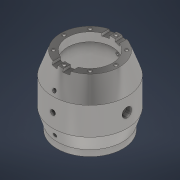
# Autodesk Inventor part: Emitter_Barrel
Saved by Autodesk Inventor 2022 (Build 260153000, 153)
## iProperties
Created: 2024-05-08
Part Number: Emitter_Barrel
Material: Generic
Document SubType Name: Modeling
Designer: jo_ki
Density: 1 g/cm^3
Appearance: Steel - Polished
Author: jo_ki
Autodesk Inventor part; units mm, degrees
sketch "Sketch1" plane through (0, 0, 0) normal (0, 0, 1) x (1, 0, 0)
  line L0 (0, 48) -> (0, -8) projected
  line L1 (0, 0) -> (19, 0)
  line L2 (19, 0) -> (19, 3.5)
  line L3 (19, 3.5) -> (21.5, 11.5)
  line L4 (21.5, 11.5) -> (21.5, 27.5)
  line L5 (21.5, 27.5) -> (17, 40)
  line L6 (17, 40) -> (13, 40)
  line L7 (13, 40) -> (13, 0)
  line L8 (-4.3, 0) -> (25.8, 0) construction
  line L9 (5.125, 40) -> (1.625, 40)
  line L10 (1.625, 40) -> (1.625, 38.5)
  line L11 (1.625, 38.5) -> (5.125, 38.5)
  line L12 (5.125, 38.5) -> (5.125, 40)
  line L13 (13, 35) -> (16, 35)
  line L14 (16, 35) -> (16, 0)
  line L15 (14, 40) -> (14, 0)
  point P0 (16, 0)
  dimension "d0" = 38
  dimension "d1" = 3.5
  dimension "d2" = 43
  dimension "d3" = 11.5
  dimension "d5" = 34
  dimension "d6" = 40
  dimension "d7" = 26
  dimension "d9" = 3.5
  dimension "d10" = 1.5
  dimension "d11" = 3.25
  dimension "d24" = 32
  dimension "d56" = 27.5
  dimension "d57" = 5
  dimension "d59" = 2
  constraints: 28 end point, 5 perpendicular, 5 point on line, 4 parallel, 3 horizontal, 1 collinear
  measures "d0" diameter of L1.end L0
  measures "d1" distance from line of L2.end L8
  measures "d2" diameter of L3.end L0
  measures "d3" distance from line of L8 L3.end
  measures "d5" diameter of L5.end L0
  measures "d6" distance from line of L8 L5.end
  measures "d7" diameter of L6.end L0
  measures "d9" distance between parallel lines of L10 L12
  measures "d10" distance between parallel lines of L11 L9
  measures "d11" diameter of L10 L0
  measures "d24" diameter of L14 L0
  measures "d56" distance from line of L8 L4.end
  measures "d57" distance between parallel lines of L13 L6
  measures "d59" distance between parallel lines of L15 L14
revolve "Revolution1" add sketch "Sketch1" angle 360 about axis through (0, 0, 0) along (0, -1, 0) contours L7 L6 L15 L13 | L14 L13 L15 L6 L5 L4 L3 L2 L1
extrude "Extrusion1" cut sketch "Sketch1" along normal through all both and the other way through all contours L12 L11 L10 L9
mirror "Mirror1" about plane through (0, 0, 0) normal (1, 0, 0) of "Extrusion1"
sketch "Sketch4" plane through (1.625, 40, 16.9222) normal (0, 1, 0) x (1, 0, 0)
  line L0 (-3.25, 4.0241) -> (-3.25, 0) projected
  arc A0 (-3.25, 0) -> (0, 0) centre (-1.625, 16.9222) ccw projected
  line L1 (0, 0) -> (0, 4.0241) projected
  arc A1 (-3.25, 4.0241) -> (0, 4.0241) centre (-1.625, 16.9222) ccw projected
  line L2 (-1.625, 3.9222) -> (-1.625, -0.0778)
  line L3 (0, 29.8202) -> (0, 33.8443) projected
  line L4 (-3.25, 33.8443) -> (-3.25, 29.8202) projected
  arc A2 (0, 33.8443) -> (-3.25, 33.8443) centre (-1.625, 16.9222) ccw projected
  arc A3 (-3.25, 4.0241) -> (0, 4.0241) centre (-1.625, 16.9222) ccw projected
  arc A4 (0, 29.8202) -> (-3.25, 29.8202) centre (-1.625, 16.9222) ccw projected
  point P0 (-1.625, 1.9222)
  constraints: 2 end point, 2 point on circle, 1 midpoint
hole "Hole1" at (0, 40, 15) direction (0, -1, 0) diameter 2 depth 0.5 tip angle 118
pattern_circular "Circular Pattern1" count 8 over 360 about axis through (0, -10, 0) along (0, 1, 0) of "Hole1"
ref_plane "Work Plane1" through (0, 19.5, 21.5) normal (0, 0, 1) x (1, 0, 0)
sketch "Sketch5" plane through (0, 19.5, 21.5) normal (0, 0, 1) x (1, 0, 0)
  line L0 (-21.5, 8) -> (21.5, 8) projected
  line L1 (-21.5, -8) -> (21.5, -8) projected
  line L2 (-21.5, -8) -> (21.5, -8) projected
  line L3 (-21.5, 8) -> (21.5, 8) projected
  line L4 (0, 8) -> (0, -8)
  point P0 (0, -19.5)
  point P1 (0, 0)
  constraints: 3 midpoint, 2 end point
hole "Hole2" at (0, 19.5, 21.5) direction (0, 0, -1) diameter 2.9 depth 7.6 clearance for "Countersunk Flat Head Screw ISO 2009/7046" size "M2.5" standard "ISO"
ref_plane "Work Plane2" through (21.5, 19.5, 0) normal (1, 0, 0) x (0, 1, 0)
sketch "Sketch6" plane through (21.5, 19.5, 0) normal (1, 0, 0) x (0, 1, 0)
  line L0 (8, 21.5) -> (8, -21.5) projected
  line L1 (-8, 21.5) -> (-8, -21.5) projected
  line L2 (8, 0) -> (-8, 0)
  point P0 (-19.5, 0)
  point P1 (0, 0)
  constraints: 3 midpoint, 2 end point
hole "Hole3" at (21.5, 19.5, 0) direction (-1, 0, 0) diameter 2.9 depth 10 counterbore diameter 5.5 counterbore depth 2.9 clearance for "Socket Head Cap Screw DIN EN ISO 4762" size "M2.5" standard "DIN"
mirror "Mirror2" about plane through (0, 0, 0) normal (1, 0, 0) of "Hole3"
ref_plane "Work Plane3" through (0, 19.5, 21.5) normal (0, 0, 1) x (1, 0, 0)
sketch "Sketch7" plane through (0, 19.5, 21.5) normal (0, 0, 1) x (1, 0, 0)
  line L0 (-21.5, -8) -> (21.5, -8) projected
  line L1 (-19, -16) -> (19, -16) projected
  line L2 (-21.5, -8) -> (21.5, -8) projected
  line L3 (0, -8) -> (0, -16)
  line L4 (-21.5, 8) -> (21.5, 8) projected
  line L5 (-1.625, 20.5) -> (-1.625, 19) projected
  line L6 (-1.625, 19) -> (-5.125, 19) projected
  line L7 (-5.125, 19) -> (-5.125, 20.5) projected
  line L8 (-5.125, 20.5) -> (-5.125, 20.5) projected
  line L9 (-5.125, 20.5) -> (-5.125, 19) projected
  line L10 (-5.125, 19) -> (-1.625, 19) projected
  line L11 (-1.625, 19) -> (-1.625, 20.5) projected
  line L12 (-1.625, 20.5) -> (1.625, 20.5) projected
  line L13 (1.625, 20.5) -> (1.625, 19) projected
  line L14 (1.625, 19) -> (5.125, 19) projected
  line L15 (5.125, 19) -> (5.125, 20.5) projected
  line L16 (5.125, 20.5) -> (5.125, 20.5) projected
  line L17 (5.125, 20.5) -> (5.125, 19) projected
  line L18 (5.125, 19) -> (1.625, 19) projected
  line L19 (1.625, 19) -> (1.625, 20.5) projected
  line L20 (1.625, 20.5) -> (-1.625, 20.5) projected
  line L21 (-1.625, 20.5) -> (1.625, 20.5) projected
  line L22 (0, 20.5) -> (0, 8)
  point P0 (0, -19.5)
  point P1 (0, -12)
  point P2 (0, 10.5)
  dimension "d58" = 10
  constraints: 5 midpoint, 4 end point, 1 point on line
  measures "d58" distance of L22.start point (0, 10.5)
hole "Hole4" at (0, 7.5, 21.5) at (0, 30, 21.5) direction (0, 0, -1) diameter 2.013 depth 20 thread size "M2.5x0.45" class "6H" standard "ISO Metric profile"
pattern_circular "Circular Pattern3" count 2 over 360 about axis through (0, -10, 0) along (0, 1, 0) of "Hole4"
equation "\"d47\" = d58"
body "Solid1"
